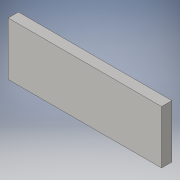
# Autodesk Inventor part: RTS Board
Saved by Autodesk Inventor 2016 (Build 200138000, 138)
## iProperties
Created: 2016-10-07
Part Number: RTS Board
Material: Generic
Document SubType Name: Modeling
Designer: sullir
Density: 1 g/cm^3
Appearance: Default
Author: sullir
Autodesk Inventor part; units mm, degrees
ref_plane "YZ Plane" through (0, 0, 0) normal (1, 0, 0) x (0, 1, 0)
ref_plane "XZ Plane" through (0, 0, 0) normal (0, 1, 0) x (-1, 0, 0)
ref_plane "XY Plane" through (0, 0, 0) normal (0, 0, 1) x (1, 0, 0)
sketch "Sketch1" plane through (0, 0, 0) normal (0, 0, 1) x (1, 0, 0)
  line L0 (-74.903, -67.9207) -> (85.117, -67.9207)
  line L1 (85.117, -67.9207) -> (85.117, -123.4197)
  line L2 (85.117, -123.4197) -> (-74.903, -123.4197)
  line L3 (-74.903, -123.4197) -> (-74.903, -67.9207)
  point P0 (0, 0)
  dimension "d0" = 160.02
  dimension "d1" = 55.499
  constraints: 8 end point, 2 parallel, 1 horizontal, 1 perpendicular
  measures "d0" distance of L0.start L0.end
  measures "d1" distance between parallel lines of L0 L2
extrude "Extrusion1" add sketch "Sketch1" along normal blind 10.7442
body "Solid1"
